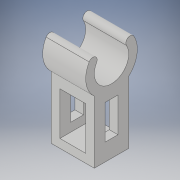
# Autodesk Inventor part: Thread_Clip
Saved by Autodesk Inventor 2019 (Build 230136000, 136)
## iProperties
Created: 2019-11-14
Part Number: Thread_Clip
Material: Generic
Document SubType Name: Modeling
Designer: James
Density: 1 g/cm^3
Appearance: Default
Author: James
Autodesk Inventor part; units mm, degrees
ref_plane "YZ Plane" through (0, 0, 0) normal (1, 0, 0) x (0, 1, 0)
ref_plane "XZ Plane" through (0, 0, 0) normal (0, 1, 0) x (-1, 0, 0)
ref_plane "XY Plane" through (0, 0, 0) normal (0, 0, 1) x (1, 0, 0)
sketch "Sketch1" plane through (0, 0, 0) normal (1, 0, 0) x (0, 1, 0)
  arc A0 (2, 3.4641) -> (2, -3.4641) centre (0, 0) ccw
  arc A1 (2, 3.4641) -> (3, 5.1962) centre (2.5, 4.3301) ccw
  arc A2 (3, -5.1962) -> (2, -3.4641) centre (2.5, -4.3301) ccw
  line L0 (-4.4721, 4) -> (-19, 4)
  line L1 (-19, 4) -> (-19, -4)
  line L2 (-19, -4) -> (-4.4721, -4)
  arc A3 (3, 5.1962) -> (-4.4721, 4) centre (0, 0) ccw
  arc A4 (-4.4721, -4) -> (3, -5.1962) centre (0, 0) ccw
  point P0 (-6, 0)
  point P1 (-19, 0)
  dimension "d0" = 8
  dimension "d2" = 2.5
  dimension "d3" = 8
  dimension "d6" = 19
  dimension "d7" = 6
  dimension "d8" = 6
  constraints: 10 point on circle, 6 end point, 5 centre point, 3 tangent, 2 coincident, 1 equal radius, 1 horizontal, 1 horizontal alignment, 1 midpoint, 1 parallel, 1 perpendicular, 1 vertical alignment
  measures "d0" diameter of A0
  measures "d2" horizontal distance of point (0, 0) A1.centre
  measures "d3" distance of L0.end L1.end
  measures "d6" distance from line of point (0, 0) L1
  measures "d7" radius of A3
  measures "d8" radius of A4
extrude "Extrusion1" add sketch "Sketch1" along normal blind 10
sketch "Sketch2" plane through (0, -19, 4) normal (0, 0, 1) x (1, 0, 0)
  line L0 (2, 12) -> (8, 12)
  line L1 (8, 12) -> (8, 2)
  line L2 (8, 2) -> (2, 2)
  line L3 (2, 2) -> (2, 12)
  line L4 (0, 0) -> (10, 0) projected
  line L5 (10, 14.5279) -> (10, 0) projected
  point P0 (0, 19)
  dimension "d11" = 2
  dimension "d12" = 6
  dimension "d13" = 10
  dimension "d14" = 2
  constraints: 8 end point, 2 parallel, 1 horizontal, 1 perpendicular
  measures "d11" distance between parallel lines of L4 L2
  measures "d12" distance of L1.end L2.end
  measures "d13" distance of L0.end L1.end
  measures "d14" distance between parallel lines of L5 L1
extrude "Extrusion2" cut sketch "Sketch2" against normal blind 10
sketch "Sketch3" plane through (0, 0, 0) normal (-1, 0, 0) x (0, 0, 1)
  line L0 (-1.5, -7) -> (1.5, -7)
  line L1 (1.5, -7) -> (1.5, -15)
  line L2 (1.5, -15) -> (-1.5, -15)
  line L3 (-1.5, -15) -> (-1.5, -7)
  line L4 (4, -7) -> (-4, -7) projected
  line L5 (4, -17) -> (-4, -17) projected
  line L6 (4, -4.4721) -> (4, -19) projected
  point P0 (0, 0)
  point P1 (0, -7)
  point P2 (0, -7)
  dimension "d17" = 3
  dimension "d18" = 2
  dimension "d19" = 2.5
  constraints: 8 end point, 2 midpoint, 2 parallel, 1 coincident, 1 horizontal, 1 perpendicular
  measures "d17" distance of L1.end L2.end
  measures "d18" distance between parallel lines of L5 L2
  measures "d19" distance between parallel lines of L6 L1
extrude "Extrusion3" cut sketch "Sketch3" against normal blind 10
body "Solid1"
